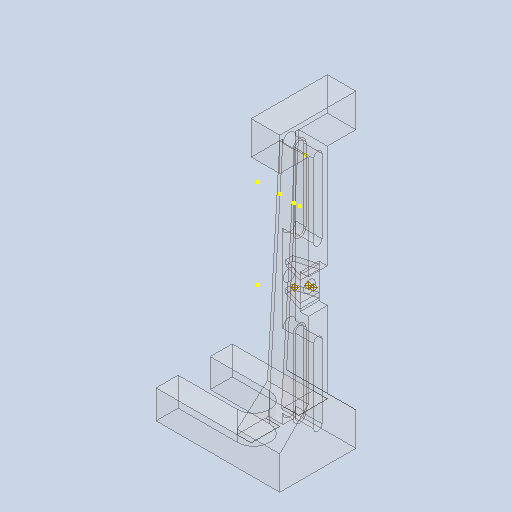
# Autodesk Inventor part: acrylic_side_holder_plunger2
Saved by Autodesk Inventor 2025 (Build 290162000, 162)
## iProperties
Created: 2024-04-25
Part Number: acrylic_side_holder_plunger2
Material: Acetal Resin, Black
Document SubType Name: Modeling
Designer: warke
Density: 1.425 g/cm^3
Appearance: Smooth - Black
Mass: 4.59418 g
Surface Area: 36.0835 cm^2
Volume: 3.82848 cm^3
Author: warke
Autodesk Inventor part; units mm, degrees
ref_plane "YZ Plane" through (0, 0, 0) normal (1, 0, 0) x (0, 1, 0)
ref_plane "XZ Plane" through (0, 0, 0) normal (0, 1, 0) x (-1, 0, 0)
ref_plane "XY Plane" through (0, 0, 0) normal (0, 0, 1) x (1, 0, 0)
sketch "Sketch1" plane through (0, 0, 0) normal (0, 0, 1) x (1, 0, 0)
  line L0 (8, -18.45) -> (8, -12.75)
  line L1 (7.5, -23.7) -> (7.5, -41.2)
  line L2 (7.5, -18.7) -> (7.5, -23.7)
  line L3 (7.5, -7.5) -> (7.5, -12.5)
  line L4 (7.5, 10) -> (7.5, -7.5)
  line L5 (7.5, 15) -> (7.5, 10)
  line L6 (7.5, -41.2) -> (7.5, -46.2)
  line L7 (8.5, -18.45) -> (8.5, -12.5)
  line L8 (8.5, -12.5) -> (7.5, -12.5)
  line L9 (8.5, -18.45) -> (8.5, -18.7)
  line L10 (8.5, -18.7) -> (7.5, -18.7)
  line L11 (7.5, -46.2) -> (10.5, -46.2)
  line L12 (10.5, -46.2) -> (10.5, 15)
  line L13 (10.5, 15) -> (7.5, 15)
  point P0 (0, 0)
extrude "Extrusion1" add sketch "Sketch1" against normal blind 4
sketch "Sketch2" plane through (7.5, -46.2, 0) normal (-1, 0, 0) x (0, 0, 1)
  line L0 (0, 61.2) -> (-4, 61.2) projected
  arc A0 (-1.111, 55.2) -> (-2.889, 55.2) centre (-2, 55.2) ccw
  arc A1 (-2.889, 39.7) -> (-1.111, 39.7) centre (-2, 39.7) ccw
  line L1 (-2.889, 55.2) -> (-2.889, 39.7)
  line L2 (-1.111, 39.7) -> (-1.111, 55.2)
  line L3 (-2, 55.2) -> (-2, 54.311)
  line L4 (-2, 40.589) -> (-2, 39.7)
  line L5 (0, 0) -> (-4, 0) projected
  arc A2 (-1.111, 55.2) -> (-2.889, 55.2) centre (-2, 55.2) ccw
  arc A3 (-2.889, 39.7) -> (-1.111, 39.7) centre (-2, 39.7) ccw
  line L6 (-2.889, 55.2) -> (-2.889, 39.7)
  line L7 (-1.111, 39.7) -> (-1.111, 55.2)
  line L8 (-2, 55.2) -> (-2, 54.311)
  line L9 (-2, 40.589) -> (-2, 39.7)
  arc A4 (-1.111, 21.5) -> (-2.889, 21.5) centre (-2, 21.5) ccw
  arc A5 (-2.889, 6) -> (-1.111, 6) centre (-2, 6) ccw
  line L10 (-2.889, 21.5) -> (-2.889, 6)
  line L11 (-1.111, 6) -> (-1.111, 21.5)
  line L12 (-2, 21.5) -> (-2, 20.611)
  line L13 (-2, 6.889) -> (-2, 6)
  line L14 (-2.889, 21.5) -> (-2.889, 6)
  line L15 (-1.111, 6) -> (-1.111, 21.5)
  line L16 (-2, 21.5) -> (-2, 20.611)
  arc A6 (-1.111, 21.5) -> (-2.889, 21.5) centre (-2, 21.5) ccw
  arc A7 (-2.889, 6) -> (-1.111, 6) centre (-2, 6) ccw
  line L17 (-2, 6.889) -> (-2, 6)
  point P0 (0, 46.2)
  point P1 (-2, 39.7)
  point P2 (-2, 6)
  point P3 (-1.111, 21.5)
  point P4 (-2.889, 21.5)
  dimension "d5" = 1.778
  dimension "d6" = 15.5
  dimension "d7" = 1.778
  dimension "d9" = 1.778
  dimension "d10" = 15.5
  dimension "d11" = 1.778
  dimension "d12" = 1.778
  dimension "d13" = 15.5
  dimension "d14" = 1.778
  dimension "d15" = 1.778
  dimension "d16" = 15.5
  dimension "d17" = 1.778
  constraints: 32 end point, 16 point on circle, 12 vertical, 8 centre point, 8 tangent, 7 coincident
  measures "d5" diameter of A0
  measures "d6" distance of L4.end L3.start
  measures "d7" diameter of A1
  measures "d9" diameter of A2
  measures "d10" distance of L8.start L4.end
  measures "d11" diameter of A3
  measures "d12" diameter of A4
  measures "d13" distance of L13.end L12.start
  measures "d14" diameter of A5
  measures "d15" diameter of A6
  measures "d16" distance of L16.start L13.end
  measures "d17" diameter of A7
sketch "Sketch3" plane through (7.5, -12.5, 0) normal (-1, 0, 0) x (0, 0, 1)
  arc A0 (-0.65, 21.5) -> (-3.35, 21.5) centre (-2, 21.5) ccw
  arc A1 (-3.35, 6) -> (-0.65, 6) centre (-2, 6) ccw
  line L0 (-0.65, 21.5) -> (-0.65, 6)
  line L1 (-3.35, 6) -> (-3.35, 21.5)
  arc A2 (-0.65, -12.2) -> (-3.35, -12.2) centre (-2, -12.2) ccw
  arc A3 (-3.35, -27.7) -> (-0.65, -27.7) centre (-2, -27.7) ccw
  line L2 (-0.65, -12.2) -> (-0.65, -27.7)
  line L3 (-3.35, -27.7) -> (-3.35, -12.2)
  point P0 (0, 12.5)
  point P1 (-2, -12.2)
  dimension "d30" = 2.7
  dimension "d31" = 2.7
  dimension "d32" = 2.7
  dimension "d33" = 2.7
  constraints: 8 end point, 8 point on circle, 4 centre point, 4 tangent, 2 coincident, 2 vertical
  measures "d30" diameter of A0
  measures "d31" diameter of A1
  measures "d32" diameter of A2
  measures "d33" diameter of A3
extrude "Extrusion2" cut sketch "Sketch2" against normal through all
extrude "Extrusion3" cut sketch "Sketch3" against normal blind 1.7
sketch "Sketch4" plane through (8.5, -18.7, 0) normal (-1, 0, 0) x (0, 0, 1)
  line L0 (0, 6.2) -> (0, 0) projected
  line L1 (0, 6.2) -> (-4, 6.2) projected
  line L2 (-4, 0) -> (-4, 6.2) projected
  line L3 (0, 0) -> (-4, 0) projected
  point P0 (0, 18.7)
extrude "Extrusion4" cut sketch "Sketch4" against normal through all
sketch "Sketch5" plane through (7.5, -12.5, 0) normal (-1, 0, 0) x (0, 0, 1)
  line L0 (0, -6.2) -> (-4, -6.2) projected
  line L1 (0, 0) -> (-4, 0)
  line L2 (-4, 0) -> (-4, -6.2)
  line L3 (-4, -6.2) -> (0, -6.2)
  line L4 (0, -6.2) -> (0, 0)
  point P0 (0, 12.5)
  constraints: 8 end point, 2 parallel, 1 horizontal, 1 perpendicular
extrude "Extrusion5" add sketch "Sketch5" against normal blind 2
hole "Hole1" at (9.5, -15.6, -2) direction (-1, 0, 0) diameter 2.5 end through all
sketch "Sketch6" plane through (7.5, -46.2, 0) normal (-1, 0, 0) x (0, 0, 1)
  circle A0 centre (-2, 30.6) radius 1.25 projected
  arc A1 (-0.65, 55.2) -> (-3.35, 55.2) centre (-2, 55.2) ccw projected
  line L0 (-0.65, 55.2) -> (-0.65, 39.7) projected
  arc A2 (-3.35, 39.7) -> (-0.65, 39.7) centre (-2, 39.7) ccw projected
  line L1 (-3.35, 39.7) -> (-3.35, 55.2) projected
  arc A3 (-0.65, 21.5) -> (-3.35, 21.5) centre (-2, 21.5) ccw projected
  line L2 (-0.65, 21.5) -> (-0.65, 6) projected
  arc A4 (-3.35, 6) -> (-0.65, 6) centre (-2, 6) ccw projected
  line L3 (-3.35, 6) -> (-3.35, 21.5) projected
  line L4 (0, 61.2) -> (0, 0) projected
  line L5 (0, 61.2) -> (-4, 61.2) projected
  line L6 (-4, 0) -> (-4, 61.2) projected
  line L7 (0, 0) -> (-4, 0) projected
  line L8 (0, 33.7) -> (-4, 33.7) projected
  line L9 (-4, 27.5) -> (0, 27.5) projected
  line L10 (0, 33.7) -> (-1.25, 33.7)
  line L11 (-1.25, 33.7) -> (-2.75, 33.7)
  line L12 (-2.75, 33.7) -> (-2.75, 32.7)
  line L13 (-2.75, 32.7) -> (-1.25, 32.7)
  line L14 (-1.25, 32.7) -> (-1.25, 33.7)
  line L15 (-1.25, 27.5) -> (-2.75, 27.5)
  line L16 (-2.75, 27.5) -> (-2.75, 28.5)
  line L17 (-2.75, 28.5) -> (-1.25, 28.5)
  line L18 (-1.25, 28.5) -> (-1.25, 27.5)
  point P0 (0, 46.2)
  point P1 (-2.75, 27.5)
  dimension "d53" = 1.25
  dimension "d54" = 1.5
  dimension "d55" = 1
  dimension "d56" = 1
  constraints: 18 end point, 4 parallel, 2 horizontal, 2 perpendicular, 2 point on line
  measures "d53" distance of L8.start L10.end
  measures "d54" distance of L13.end L12.end
  measures "d55" distance of L12.end L11.end
  measures "d56" distance of L15.end L16.end
extrude "Extrusion6" cut sketch "Sketch6" along normal mid plane 20 contours L14 L13 L12 L8 | L9 L16 L17 L18
sketch "Sketch7" plane through (7.5, -46.2, 0) normal (-1, 0, 0) x (0, 0, 1)
  point P0 (0, 46.2)
sketch "Sketch8" plane through (7.5, -46.2, 0) normal (-1, 0, 0) x (0, 0, 1)
  circle A0 centre (-2, 30.6) radius 1.25 projected
  arc A1 (-0.65, 55.2) -> (-3.35, 55.2) centre (-2, 55.2) ccw projected
  line L0 (-0.65, 55.2) -> (-0.65, 39.7) projected
  arc A2 (-3.35, 39.7) -> (-0.65, 39.7) centre (-2, 39.7) ccw projected
  line L1 (-3.35, 39.7) -> (-3.35, 55.2) projected
  arc A3 (-0.65, 21.5) -> (-3.35, 21.5) centre (-2, 21.5) ccw projected
  line L2 (-0.65, 21.5) -> (-0.65, 6) projected
  arc A4 (-3.35, 6) -> (-0.65, 6) centre (-2, 6) ccw projected
  line L3 (-3.35, 6) -> (-3.35, 21.5) projected
  line L4 (0, 61.2) -> (0, 0) projected
  line L5 (0, 61.2) -> (-4, 61.2) projected
  line L6 (-4, 0) -> (-4, 61.2) projected
  line L7 (0, 0) -> (-4, 0) projected
  point P0 (0, 46.2)
extrude "Extrusion7" add sketch "Sketch8" along normal blind 3
sketch "Sketch10" plane through (0, 0, 0) normal (0, 0, 1) x (1, 0, 0)
  line L0 (4.5, 15) -> (4.5, -46.2) projected
  line L1 (4.5, -15.6) -> (10.5, -15.6)
  line L2 (10.5, -12.5) -> (10.5, 15) projected
  line L3 (4.5, -30.6) -> (10.5, -30.6)
  line L4 (10.5, -30.6) -> (10.5, -0.6)
  line L5 (10.5, -0.6) -> (4.5, -0.6)
  line L6 (4.5, -0.6) -> (4.5, -30.6)
  line L7 (4.5, -30.6) -> (10.5, -0.6) construction
  line L8 (10.5, -30.6) -> (4.5, -0.6) construction
  line L9 (2.5, -33.1) -> (2.5, -28.1)
  line L10 (2.5, -28.1) -> (6.5, -28.1)
  line L11 (6.5, -28.1) -> (6.5, -33.1)
  line L12 (6.5, -33.1) -> (2.5, -33.1)
  line L13 (2.5, -33.1) -> (6.5, -28.1) construction
  line L14 (2.5, -28.1) -> (6.5, -33.1) construction
  line L15 (2.5, -3.1) -> (2.5, 1.9)
  line L16 (2.5, 1.9) -> (6.5, 1.9)
  line L17 (6.5, 1.9) -> (6.5, -3.1)
  line L18 (6.5, -3.1) -> (2.5, -3.1)
  line L19 (2.5, -3.1) -> (6.5, 1.9) construction
  line L20 (2.5, 1.9) -> (6.5, -3.1) construction
  line L21 (4.5, -33.1) -> (4.5, -28.1)
  line L22 (4.5, -3.1) -> (4.5, 1.9)
  line L23 (4.5, -33.1) -> (4.5, -28.1)
  point P0 (0, 0)
  point P1 (7.5, -15.6)
  point P2 (4.5, -3.1)
  point P3 (4.5, -33.1)
  point P4 (4.5, -28.1)
  dimension "d74" = 30
  dimension "d75" = 5
  dimension "d76" = 4
  dimension "d77" = 5
  constraints: 44 end point, 12 midpoint, 6 parallel, 3 perpendicular, 2 horizontal, 1 collinear, 1 point on line
  measures "d74" distance of L4.end L3.end
  measures "d75" distance of L9.start L9.end
  measures "d76" distance of L9.end L10.end
  measures "d77" distance of L15.start L15.end
extrude "Extrusion8" [suppressed]
sketch "Sketch11" plane through (10.5, 15, 0) normal (0, 1, 0) x (1, 0, 0)
  line L0 (0, 0) -> (-6, 0) projected
  line L1 (0, 0) -> (0, 4) projected
  line L2 (0, 4) -> (-6, 4) projected
  line L3 (-6, 0) -> (-6, 4) projected
  point P0 (-10.5, 0)
extrude "Extrusion9" add sketch "Sketch11" along normal blind 1.8
sketch "Sketch12" plane through (0, 0, -4) normal (0, 0, -1) x (-1, 0, 0)
  line L0 (-10.5, -12.5) -> (-10.5, 16.8) projected
  line L1 (-4.5, 16.8) -> (-10.5, 16.8)
  line L2 (-10.5, 16.8) -> (-10.5, 9.8)
  line L3 (-10.5, 9.8) -> (-4.5, 9.8)
  line L4 (-4.5, 9.8) -> (-4.5, 16.8)
  point P0 (0, 0)
  dimension "d82" = 7
  constraints: 8 end point, 2 parallel, 1 horizontal, 1 perpendicular, 1 point on line
  measures "d82" distance of L2.end L1.end
extrude "Extrusion10" add sketch "Sketch12" along normal blind 6
sketch "Sketch13" plane through (4.5, -46.2, 0) normal (-1, 0, 0) x (0, 0, 1)
  point P0 (0, 46.2)
sketch "Sketch14" plane through (0, 0, -10) normal (0, 0, -1) x (-1, 0, 0)
  point P0 (0, 0)
sketch "Sketch15" plane through (0, 0, 0) normal (0, 0, 1) x (1, 0, 0)
  line L0 (4.5, -46.2) -> (4.5, 16.8) projected
  line L1 (10.5, -12.5) -> (10.5, 9.8) projected
  line L2 (4.5, 16.8) -> (10.5, 16.8)
  line L3 (10.5, 16.8) -> (10.5, 9.8)
  line L4 (10.5, 9.8) -> (4.5, 9.8)
  line L5 (4.5, 9.8) -> (4.5, 16.8)
  point P0 (0, 0)
  constraints: 8 end point, 2 parallel, 1 horizontal, 1 perpendicular
extrude "Extrusion11" add sketch "Sketch15" along normal blind 6
sketch "Sketch16" plane through (9.2, -12.5, 0) normal (-1, 0, 0) x (0, 0, 1)
  arc A0 (-2.889, -27.7) -> (-1.111, -27.7) centre (-2, -27.7) ccw projected
  line L0 (-2.889, -12.2) -> (-2.889, -27.7) projected
  arc A1 (-1.111, -12.2) -> (-2.889, -12.2) centre (-2, -12.2) ccw projected
  line L1 (-1.111, -27.7) -> (-1.111, -12.2) projected
  line L2 (-0.65, -12.2) -> (-0.65, -27.7) projected
  arc A2 (-0.65, -12.2) -> (-3.35, -12.2) centre (-2, -12.2) ccw projected
  line L3 (-3.35, -27.7) -> (-3.35, -12.2) projected
  arc A3 (-3.35, -27.7) -> (-0.65, -27.7) centre (-2, -27.7) ccw projected
  line L4 (-1.111, 6) -> (-1.111, 21.5) projected
  arc A4 (-2.889, 6) -> (-1.111, 6) centre (-2, 6) ccw projected
  line L5 (-2.889, 21.5) -> (-2.889, 6) projected
  arc A5 (-1.111, 21.5) -> (-2.889, 21.5) centre (-2, 21.5) ccw projected
  line L6 (-0.65, 21.5) -> (-0.65, 6) projected
  arc A6 (-0.65, 21.5) -> (-3.35, 21.5) centre (-2, 21.5) ccw projected
  line L7 (-3.35, 6) -> (-3.35, 21.5) projected
  arc A7 (-3.35, 6) -> (-0.65, 6) centre (-2, 6) ccw projected
  point P0 (0, 12.5)
extrude "Extrusion12" add sketch "Sketch16" along normal blind 2.54
sketch "Sketch17" plane through (10.5, -46.2, -4) normal (0, -1, 0) x (1, 0, 0)
  line L0 (-6, 4) -> (0, 4) projected
  line L1 (-6, 0) -> (-6, 4) projected
  line L2 (0, 0) -> (-6, 0) projected
  line L3 (0, 4) -> (0, 0) projected
  point P0 (-10.5, 4)
extrude "Extrusion13" add sketch "Sketch17" along normal blind 2
sketch "Sketch18" plane through (0, 0, 0) normal (0, 0, 1) x (1, 0, 0)
  line L0 (10.5, -48.2) -> (10.5, -18.7) projected
  line L1 (4.5, -48.2) -> (10.5, -48.2)
  line L2 (10.5, -48.2) -> (10.5, -41.2)
  line L3 (10.5, -41.2) -> (4.5, -41.2)
  line L4 (4.5, -41.2) -> (4.5, -48.2)
  point P0 (0, 0)
  dimension "d91" = 7
  constraints: 8 end point, 2 parallel, 1 horizontal, 1 perpendicular, 1 point on line
  measures "d91" distance of L2.end L1.end
extrude "Extrusion14" add sketch "Sketch18" along normal blind 6
sketch "Sketch19" plane through (0, 0, -4) normal (0, 0, -1) x (-1, 0, 0)
  line L0 (-4.5, -48.2) -> (-10.5, -48.2) projected
  line L1 (-10.5, -18.7) -> (-10.5, -48.2) projected
  line L2 (-4.5, -48.2) -> (-10.5, -48.2)
  line L3 (-10.5, -48.2) -> (-10.5, -41.2)
  line L4 (-10.5, -41.2) -> (-4.5, -41.2)
  line L5 (-4.5, -41.2) -> (-4.5, -48.2)
  point P0 (0, 0)
  dimension "d94" = 7
  constraints: 8 end point, 2 parallel, 1 horizontal, 1 perpendicular, 1 point on line
  measures "d94" distance of L2.end L3.end
extrude "Extrusion15" add sketch "Sketch19" along normal blind 6
sketch "Sketch21" plane through (4.5, -46.2, 0) normal (-1, 0, 0) x (0, 0, 1)
  line L0 (-10, -2) -> (6, -2) projected
  line L1 (-10, -2) -> (6, -2)
  line L2 (6, -2) -> (6, 5)
  line L3 (6, 5) -> (-10, 5)
  line L4 (-10, 5) -> (-10, -2)
  point P0 (0, 46.2)
  constraints: 8 end point, 2 parallel, 1 horizontal, 1 perpendicular
extrude "Extrusion16" add sketch "Sketch21" along normal blind 20
sketch "Sketch22" plane through (4.5, -41.2, 0) normal (0, 1, 0) x (1, 0, 0)
  line L0 (-20, -6) -> (-20, 10) projected
  line L1 (-20, 2) -> (-7.5, 2)
  circle A0 centre (-7.5, 2) radius 3.3782
  line L2 (-7.5, 5.3782) -> (-20, 5.3782)
  line L3 (-7.5, -1.3782) -> (-20, -1.3782)
  point P0 (-4.5, 0)
  dimension "d111" = 12.5
  dimension "d112" = 6.7564
  constraints: 6 end point, 2 perpendicular, 2 point on circle, 2 point on line, 1 centre point, 1 coincident, 1 horizontal, 1 midpoint, 1 tangent
  measures "d111" distance of L1.start L1.end
  measures "d112" diameter of A0
extrude "Extrusion17" cut sketch "Sketch22" against normal through all
chamfer "Chamfer1" distance 6 angle 45 2 edges at (7.5, -41.2, -4) (7.5, -41.2, 0)
sketch "Sketch23" plane through (4.5, -41.2, -1.0931) normal (0, 1, 0) x (1, 0, 0)
  line L0 (0, -7.0931) -> (-20, -7.0931) projected
  line L1 (0, 8.9069) -> (-20, 8.9069) projected
  line L2 (-20, -7.0931) -> (-20, -2.4713) projected
  line L3 (0, 0) -> (0, -7.0931) projected
  line L4 (0, 0) -> (0, 1.8138) projected
  line L5 (-7.5, -2.4713) -> (-20, -2.4713) projected
  line L6 (-20, 4.2851) -> (-20, 8.9069) projected
  line L7 (-20, 4.2851) -> (-7.5, 4.2851) projected
  arc A0 (-7.5, -2.4713) -> (-7.5, 4.2851) centre (-7.5, 0.9069) ccw projected
  line L8 (0, 8.9069) -> (0, 1.8138) projected
  point P0 (-4.5, -1.0931)
extrude "Extrusion18" cut sketch "Sketch23" against normal blind 1
sketch "Sketch25" plane through (0, 0, -4) normal (0, 0, -1) x (-1, 0, 0)
  line L0 (-4.5, -42.2) -> (-1.5, -42.2)
  line L1 (3, -42.2) -> (-0.3782, -42.2) projected
  line L2 (-4.5, -35.2) -> (-4.5, 9.8) projected
  line L3 (-1.5, -42.2) -> (-4.5, 9.8)
  line L4 (-4.5, 9.8) -> (-4.5, -42.2)
  point P0 (0, 0)
  point P1 (-4.5, -41.2)
  dimension "d120" = 3
  constraints: 6 end point, 2 collinear
  measures "d120" distance of L0.start L0.end
extrude "Extrusion19" add sketch "Sketch25" against normal up to surface (0.65 mm away)
sketch "Sketch26" plane through (0, 0, 0) normal (0, 0, 1) x (1, 0, 0)
  line L0 (4.5, -42.2) -> (1.5, -42.2) projected
  line L1 (4.5, 9.8) -> (1.5, -42.2) projected
  line L2 (4.5, 9.8) -> (4.5, 16.8) projected
  line L3 (4.5, 9.8) -> (4.5, -42.2)
  point P0 (0, 0)
  constraints: 2 end point, 1 collinear
extrude "Extrusion20" add sketch "Sketch26" against normal up to surface (0.65 mm away)
sketch "Sketch27" plane through (4.5, -46.2, 0) normal (-1, 0, 0) x (0, 0, 1)
  line L0 (-10, 5) -> (-10, -2) projected
  line L1 (-10, 4.0073) -> (-10, 5)
  line L2 (-4, 11) -> (-10, 5) projected
  line L3 (-10, 5) -> (-4, 11)
  line L4 (-4, 11) -> (-4, 4.0073)
  line L5 (-4, 4.0073) -> (-10, 4.0073)
  line L6 (6, 5) -> (0, 11) projected
  line L7 (-0.5466, 11) -> (0, 11)
  line L8 (0, 11) -> (6, 5)
  line L9 (6, 5) -> (6, 4.0073)
  line L10 (6, 4.0073) -> (0, 4.0073)
  line L11 (0, 4.0073) -> (0, 11)
  point P0 (0, 46.2)
  constraints: 18 end point, 3 collinear, 3 point on line, 2 perpendicular, 1 horizontal, 1 parallel
extrude "Extrusion21" add sketch "Sketch27" along normal up to surface surface through (4.5, 9.8, -4) normal (-0.9983399, 0.0575965, 0)
sketch "Sketch30" plane through (4.5, -46.2, 0) normal (-1, 0, 0) x (0, 0, 1)
  circle A0 centre (-2, 30.6) radius 1.25 projected
  line L0 (-1.25, 32.7) -> (-2.75, 32.7) projected
  line L1 (-1.25, 33.7) -> (-1.25, 32.7) projected
  line L2 (-2.75, 33.7) -> (-1.25, 33.7) projected
  line L3 (-2.75, 32.7) -> (-2.75, 33.7) projected
  line L4 (-2.75, 27.5) -> (-2.75, 28.5) projected
  line L5 (-2.75, 28.5) -> (-1.25, 28.5) projected
  line L6 (-1.25, 28.5) -> (-1.25, 27.5) projected
  line L7 (-1.25, 27.5) -> (-2.75, 27.5) projected
  point P0 (0, 46.2)
extrude "Extrusion22" cut sketch "Sketch30" along normal up to surface surface through (4.5, 9.8, -4) normal (-0.9983399, 0.0575965, 0)
sketch "Sketch31" plane through (4.5, -46.2, 0) normal (-1, 0, 0) x (0, 0, 1)
  line L0 (0, 56) -> (0, 5) projected
  line L1 (-4, 23.1) -> (0, 23.1)
  line L2 (0, 23.1) -> (0, 38.1)
  line L3 (0, 38.1) -> (-4, 38.1)
  line L4 (-4, 38.1) -> (-4, 23.1)
  circle A0 centre (-2, 30.6) radius 1.25 projected
  line L5 (-4, 23.1) -> (0, 38.1) construction
  line L6 (0, 23.1) -> (-4, 38.1) construction
  point P0 (0, 46.2)
  dimension "d130" = 15
  constraints: 12 end point, 2 midpoint, 2 parallel, 1 horizontal, 1 perpendicular, 1 point on line
  measures "d130" distance of L2.end L1.end
extrude "Extrusion23" [suppressed]
sketch "Sketch33" plane through (-5.5, -46.2, 0) normal (-1, 0, 0) x (0, 0, 1)
  line L0 (-4, 23.1) -> (0, 23.1) projected
  line L1 (0, 23.1) -> (0, 38.1) projected
  line L2 (0, 38.1) -> (-4, 38.1) projected
  line L3 (-4, 38.1) -> (-4, 23.1) projected
  circle A0 centre (-2, 30.6) radius 1.25 projected
  circle A1 centre (-2, 30.6) radius 1.25 projected
  line L4 (-9.5, 23.1) -> (5.5, 23.1)
  line L5 (5.5, 23.1) -> (5.5, 38.1)
  line L6 (5.5, 38.1) -> (-9.5, 38.1)
  line L7 (-9.5, 38.1) -> (-9.5, 23.1)
  line L8 (-9.5, 23.1) -> (5.5, 38.1) construction
  line L9 (5.5, 23.1) -> (-9.5, 38.1) construction
  point P0 (0, 46.2)
  dimension "d140" = 15
  constraints: 12 end point, 2 midpoint, 2 parallel, 1 horizontal, 1 perpendicular
  measures "d140" distance of L6.end L5.end
extrude "Extrusion25" [suppressed]
hole "Hole4" [suppressed]
fillet "Fillet3" [suppressed]
sketch "Sketch34" plane through (10.5, -12.5, 0) normal (1, 0, 0) x (0, 0, -1)
  line L0 (0, 22.3) -> (0, -22.7) projected
  line L1 (4, 0.5) -> (0, 0.5)
  line L2 (0, 0.5) -> (0, -6.7)
  line L3 (0, -6.7) -> (4, -6.7)
  line L4 (4, -6.7) -> (4, 0.5)
  circle A0 centre (2, -3.1) radius 1.25 projected
  line L5 (4, 0.5) -> (0, -6.7) construction
  line L6 (0, 0.5) -> (4, -6.7) construction
  point P0 (0, 12.5)
  dimension "d155" = 7.2
  constraints: 12 end point, 2 midpoint, 2 parallel, 1 horizontal, 1 perpendicular, 1 point on line
  measures "d155" distance of L2.end L1.end
extrude "Extrusion26" cut sketch "Sketch34" against normal up to surface (1 mm away)
sketch "Sketch35" plane through (9.5, -12.5, 0) normal (1, 0, 0) x (0, 0, -1)
  line L0 (2.75, -1) -> (2.75, 0) projected
  line L1 (2.75, 0) -> (1.25, 0) projected
  line L2 (1.25, 0) -> (1.25, -1) projected
  line L3 (1.25, -1) -> (2.75, -1) projected
  line L4 (1.25, -5.2) -> (1.25, -6.2) projected
  line L5 (1.25, -6.2) -> (2.75, -6.2) projected
  line L6 (2.75, -6.2) -> (2.75, -5.2) projected
  line L7 (2.75, -5.2) -> (1.25, -5.2) projected
  point P0 (0, 12.5)
extrude "Extrusion27" cut sketch "Sketch35" along normal mid plane 20
sketch "Sketch36" plane through (0, 0, 0) normal (0, 0, 1) x (1, 0, 0)
  point P0 (0, 0)
sketch "Sketch37" plane through (9.5, -12.5, 0) normal (1, 0, 0) x (0, 0, -1)
  line L0 (4, 0.5) -> (4, -6.7) projected
  line L1 (0, -6.7) -> (0, 0.5) projected
  line L2 (4, 0.5) -> (0, 0.5)
  line L3 (0, 0.5) -> (0, -6.7)
  line L4 (0, -6.7) -> (4, -6.7)
  line L5 (4, -6.7) -> (4, 0.5)
  point P0 (0, 12.5)
  constraints: 8 end point, 2 parallel, 1 horizontal, 1 perpendicular
extrude "Extrusion28" cut sketch "Sketch37" against normal blind 0.75
sketch "Sketch38" plane through (4.5, -12.5, -2.75) normal (0, -1, 0) x (1, 0, 0)
  line L0 (0, 0) -> (0, 1.5) projected
  line L1 (4.25, 2.75) -> (4.25, -1.25) projected
  line L2 (0, 1.5) -> (4.25, 2.75)
  line L3 (4.25, 2.75) -> (4.25, -1.25)
  line L4 (4.25, -1.25) -> (0, 0)
  line L5 (0, 0) -> (0, 1.5)
  point P0 (-4.5, 2.75)
  constraints: 8 end point, 1 collinear, 1 parallel
extrude "Extrusion29" cut sketch "Sketch38" along normal up to surface (1 mm away)
sketch "Sketch39" plane through (4.5, -18.7, -1.25) normal (0, 1, 0) x (1, 0, 0)
  point P0 (-4.5, -1.25)
sketch "Sketch40" plane through (8.75, -12.5, 0) normal (1, 0, 0) x (0, 0, -1)
  point P0 (0, 12.5)
sketch "Sketch41" plane through (4.5, -18.7, -1.25) normal (0, 1, 0) x (1, 0, 0)
  line L0 (0, 0) -> (0, 1.5) projected
  line L1 (0, 1.5) -> (4.25, 2.75)
  line L2 (4.25, 2.75) -> (4.25, -1.25) projected
  line L3 (4.25, 2.75) -> (4.25, -1.25)
  line L4 (0, 1.5) -> (0, 0) projected
  line L5 (4.25, -1.25) -> (0, 0)
  line L6 (0, 0) -> (0, 1.5)
  point P0 (-4.5, -1.25)
  constraints: 8 end point, 2 collinear
extrude "Extrusion30" cut sketch "Sketch41" along normal up to surface (1 mm away)
body "Solid1"
